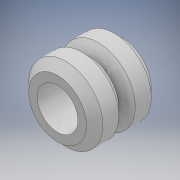
# Autodesk Inventor part: M4-608 Straight Spacer
Saved by Autodesk Inventor 2017 (Build 210142000, 142)
## iProperties
Created: 2016-04-12
Part Number: M4-608 Straight Spacer
Material: Generic
Document SubType Name: Modeling
Designer: alist
Density: 1 g/cm^3
Appearance: Default
Author: alist
## iProperties of the stored document M4-608 Straight Spacer_3DPrint.ipt
Created: 2017-01-15
Part Number: M4-608 Straight Spacer_3DPrint
Material: Generic
Document SubType Name: Modeling
Designer: Alistair
Density: 1 g/cm^3
Appearance: Default
Author: Alistair
Autodesk Inventor part; units mm, degrees
ref_plane "YZ Plane" through (0, 0, 0) normal (1, 0, 0) x (0, 1, 0)
ref_plane "XZ Plane" through (0, 0, 0) normal (0, 1, 0) x (-1, 0, 0)
sketch "Sketch1" plane through (0, 0, 0) normal (0, 1, 0) x (-1, 0, 0)
  circle A0 centre (0, 0) radius 4
  dimension "d0" = 8
  constraints: 1 centre point, 1 coincident
  measures "d0" diameter of A0
extrude "Extrusion1" add sketch "Sketch1" along normal blind 7
sketch "Sketch2" plane through (0, 7, 0) normal (0, 1, 0) x (1, 0, 0)
  circle A0 centre (0, 0) radius 5.75
  dimension "d3" = 11.5
  constraints: 1 centre point, 1 coincident
  measures "d3" diameter of A0
extrude "Extrusion2" add sketch "Sketch2" along normal blind 3.2
sketch "Sketch4" plane through (0, 0, 0) normal (1, 0, 0) x (0, 1, 0)
  line L0 (20.4, 3.1121) -> (19.5121, 4)
  line L1 (19.5121, 4) -> (17.7879, 4)
  line L2 (16.9, 3.1121) -> (17.7879, 4)
  line L3 (13.4, 3.1121) -> (14.2879, 4)
  line L4 (14.2879, 4) -> (16.0121, 4)
  line L5 (16.9, 3.1121) -> (16.0121, 4)
  line L6 (13.4, 3.1121) -> (13.4, 6.6121)
  line L7 (13.4, 8.5445) -> (20.4, 8.5445)
  line L8 (20.4, 8.5445) -> (20.4, 3.1121)
  line L9 (0, 3.1121) -> (0.8879, 4)
  line L10 (0.8879, 4) -> (2.6121, 4)
  line L11 (3.5, 3.1121) -> (2.6121, 4)
  line L12 (3.5, 3.1121) -> (4.3879, 4)
  line L13 (6.1121, 4) -> (4.3879, 4)
  line L14 (7, 3.1121) -> (6.1121, 4)
  line L15 (7, 3.1121) -> (7, 6.6121)
  line L16 (7, 8.5445) -> (0, 8.5445)
  line L17 (0, 8.5445) -> (0, 3.1121)
  line L18 (13.4, 6.6121) -> (7, 6.6121)
  line L19 (13.4, 8.5445) -> (7, 8.5445)
  line L20 (-4.08, 0) -> (24.48, 0) projected
  point P0 (0, 0)
  constraints: 40 end point, 2 perpendicular, 1 collinear, 1 parallel
revolve "Revolution1" cut sketch "Sketch4" angle 360 about axis through (0, -10, 0) along (0, 1, 0)
hole "Hole2" at (0, 0, 0) direction (0, 1, 0) diameter 4.4 end through all
ref_plane "Work Plane1" through (0, 7, 5.75) normal (0, 0, 1) x (1, 0, 0)
sketch "Sketch5" plane through (0, 7, 5.75) normal (0, 0, 1) x (1, 0, 0)
  line L0 (5.75, 3.2) -> (-5.75, 3.2) projected
  line L1 (-5.75, 0) -> (5.75, 0) projected
  line L2 (-5.75, 0) -> (-5.75, 3.2)
  line L3 (5.75, 3.2) -> (5.75, 0)
  point P0 (0, -7)
  constraints: 4 end point, 1 parallel, 1 vertical
extrude "Extrusion4" cut sketch "Sketch5" against normal through all
body "Solid1"
